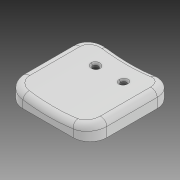
# Autodesk Inventor part: fakekeycap
Saved by Autodesk Inventor 2020 (Build 240168000, 168)
## iProperties
Created: 2020-12-13
Part Number: fakekeycap
Material: Generic
Document SubType Name: Modeling
Designer: DDeGo
Density: 1 g/cm^3
Appearance: Default
Author: DDeGo
Autodesk Inventor part; units mm, degrees
ref_plane "YZ Plane" through (0, 0, 0) normal (1, 0, 0) x (0, 1, 0)
ref_plane "XZ Plane" through (0, 0, 0) normal (0, 1, 0) x (-1, 0, 0)
ref_plane "XY Plane" through (0, 0, 0) normal (0, 0, 1) x (1, 0, 0)
sketch "Sketch1" plane through (0, 0, 0) normal (0, 0, 1) x (1, 0, 0)
  arc A0 (0, 0) -> (15, 0) centre (7.5, 29.0474) ccw
  line L0 (0, 0) -> (0, -3)
  line L1 (0, -3) -> (15, -3)
  line L2 (15, -3) -> (15, 0)
  line L3 (15, 0) -> (0, 0) construction
  dimension "d0" = 15
  dimension "d1" = 30
  dimension "d2" = 3
  constraints: 8 end point, 3 perpendicular, 2 point on circle, 1 centre point, 1 vertical
  measures "d0" distance of L2.end L0.start
  measures "d1" radius of A0
  measures "d2" distance of L1.end L2.end
extrude "Extrusion1" add sketch "Sketch1" along normal blind 15
fillet "Fillet1" radius 3 4 edges at (15, -1.5, 15) (0, -1.5, 15) (0, -1.5, 0) (15, -1.5, 0)
fillet "Fillet2" radius 1 8 edges at (14.2673, -0.1794, 13.9645) (7.5, -0.9526, 15) (0.7332, -0.1795, 13.9651) (0, 0, 7.5) (0.7332, -0.1795, 1.0349) (7.5, -0.9526, 0) (14.2673, -0.1794, 1.0355) (15, 0, 7.5)
sketch "Sketch2" plane through (3, -3, 0) normal (0, -1, 0) x (1, 0, 0)
  line L0 (0, 0) -> (9, 0) projected
  line L1 (4.5, 0) -> (4.5, 4) construction
  line L2 (4.5, 4) -> (2, 4) construction
  line L3 (4.5, 4) -> (7, 4) construction
  circle A0 centre (2, 4) radius 0.5
  circle A1 centre (7, 4) radius 0.5
  point P0 (-3, 0)
  dimension "d7" = 1
  dimension "d8" = 5
  dimension "d9" = 4
  constraints: 6 end point, 2 centre point, 2 coincident, 1 collinear, 1 equal radius, 1 horizontal, 1 midpoint, 1 perpendicular, 1 vertical
  measures "d7" diameter of A1
  measures "d8" distance of L3.end L2.end
  measures "d9" distance of L1.start L1.end
extrude "Extrusion2" cut sketch "Sketch2" against normal through all
chamfer "Chamfer1" distance 0.3 angle 45 4 edges at (9.5, -3, 4) (4.5, -3, 4) (9.5, -0.8859, 4) (4.5, -0.8022, 4)
body "Solid1"
